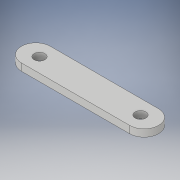
# Autodesk Inventor part: PINZA_UNION
Saved by Autodesk Inventor 2019 (Build 230136000, 136)
## iProperties
Created: 2020-02-12
Part Number: PINZA_UNION
Material: Genérico
Document SubType Name: Modeling
Designer: omar-
Density: 1 g/cm^3
Appearance: Valor por defecto
Author: omar-
Autodesk Inventor part; units mm, degrees
ref_plane "YZ Plane" through (0, 0, 0) normal (1, 0, 0) x (0, 1, 0)
ref_plane "XZ Plane" through (0, 0, 0) normal (0, 1, 0) x (-1, 0, 0)
ref_plane "XY Plane" through (0, 0, 0) normal (0, 0, 1) x (1, 0, 0)
sketch "Boceto1" plane through (0, 0, 0) normal (0, 1, 0) x (-1, 0, 0)
  circle A0 centre (14, 0) radius 1.5
  circle A1 centre (-14, 0) radius 1.5
  line L0 (15, 0) -> (-15, 0) construction
  line L1 (15, 4) -> (-15, 4)
  line L2 (-15, -4) -> (15, -4)
  arc A2 (15, -4) -> (15, 4) centre (15, 0) ccw
  arc A3 (-15, 4) -> (-15, -4) centre (-15, 0) ccw
  line L3 (0, -5.6) -> (0, 5.6) projected
  point P0 (0, 0)
  point P1 (0, 0)
  dimension "d2" = 3
  dimension "d3" = 3
  dimension "d4" = 14
  dimension "d5" = 0
  dimension "d6" = 0
  dimension "d7" = 28
  dimension "d8" = 4
  dimension "d9" = 15
  constraints: 8 end point, 4 centre point, 4 point on circle, 4 tangent, 1 coincident, 1 midpoint, 1 parallel, 1 perpendicular
  measures "d2" diameter of A0
  measures "d3" diameter of A1
  measures "d4" distance of point (0, 0) A0.centre
  measures "d5" vertical distance of point (0, 0) A0.centre
  measures "d6" vertical distance of point (0, 0) A1.centre
  measures "d7" distance of A0.centre A1.centre
  measures "d8" distance from line of point (0, 0) L2
  measures "d9" distance of point (0, 0) L0.start
extrude "Extrusión1" add sketch "Boceto1" along normal blind 2
